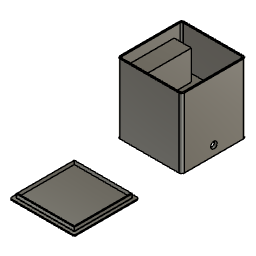
Kinderbastelprojekt, Teo der Topf, v10 (Autodesk Fusion 360 design; units mm, degrees)
part number: Kinderbastelprojekt, Teo der Topf
Autodesk Fusion 360 part; units mm, degrees
sketch "Skizze1" plane through (0, 0, 0) normal (0, 0, 1) x (1, 0, 0)
  line L0 (5, 0) -> (115, 0)
  line L1 (120, 5) -> (120, 115)
  line L2 (115, 120) -> (5, 120)
  line L3 (0, 115) -> (0, 5)
  line L4 (0, 94.8173) -> (30, 94.8173)
  line L5 (30, 94.8173) -> (30, 14.8173)
  line L6 (30, 14.8173) -> (0, 14.8173)
  line L7 (103.4005, 105.0014) -> (105.0005, 105.0014)
  line L8 (105.0005, 105.0014) -> (105.0005, 82.0014)
  line L9 (105.0005, 82.0014) -> (103.4005, 82.0014)
  line L10 (103.4005, 82.0014) -> (103.4005, 105.0014)
  arc A0 (5, 120) -> (0, 115) centre (5, 115) ccw
  arc A1 (120, 115) -> (115, 120) centre (115, 115) ccw
  arc A2 (115, 0) -> (120, 5) centre (115, 5) ccw
  arc A3 (0, 5) -> (5, 0) centre (5, 5) ccw
  point P0 (120, 0)
  point P1 (0, 120)
  dimension "d1" = 120
  dimension "d2" = 120
  dimension "d3" = 30
  dimension "d4" = 80
  dimension "d5" = 1.6
  dimension "d6" = 23
  dimension "d7" = 5
  dimension "d8" = 5
  constraint horizontal L0
  constraint vertical L1
  constraint horizontal L2
  constraint vertical L3
  constraint coincident L3 L4.start
  constraint perpendicular L3 L4
  constraint perpendicular L0 L5
  constraint perpendicular L5 L6
  constraint horizontal L7
  constraint vertical L8
  constraint horizontal L9
  constraint vertical L10
  constraint coincident P1 L2
  constraint coincident P1 L3
  constraint tangent L2 A0
  constraint tangent L3 A0
  constraint tangent L1 A1
  constraint tangent L2 A1
  constraint coincident P0 L0
  constraint coincident P0 L1
  constraint tangent L0 A2
  constraint tangent L1 A2
  constraint equal A1 A2
  constraint coincident origin L0
  constraint coincident origin L3
  constraint tangent L0 A3
  constraint tangent L3 A3
  constraint equal A1 A3
  measures "d1" distance of origin P0
  measures "d2" distance of origin P1
  measures "d3" distance of L4.start L4.end
  measures "d4" distance of L4.end L5.end
  measures "d5" distance of L7.start L7.end
  measures "d6" distance of L7.start L9.end
  measures "d7" radius of A0
  measures "d8" radius of A1
sketch "Skizze2" plane through (0, 0, 0) normal (0, 0, 1) x (1, 0, 0)
  line L0 (5, 115) -> (115, 115)
  line L1 (115, 115) -> (115, 5)
  line L2 (115, 5) -> (5, 5)
  line L3 (5, 5) -> (5, 115)
  constraint horizontal L0
  constraint perpendicular L0 L1
  constraint perpendicular L1 L2
  constraint perpendicular L0 L3
extrude "Extrusion1" add sketch "Skizze1" along normal blind 130 contours L0 L1 L2 L3 L4 L5 L6 A0 A1 A2 A3 makes body 1
extrude "Extrusion2" cut sketch "Skizze2" along normal blind 50 bodies 1
sketch "Skizze3" plane through (0, 0, 130) normal (0, 0, 1) x (-1, 0, 0)
  line L0 (-105.0005, -82.0014) -> (-103.4005, -82.0014)
  line L1 (-103.4005, -82.0014) -> (-103.4005, -105.0014)
  line L2 (-103.4005, -105.0014) -> (-105.0005, -105.0014)
  line L3 (-105.0005, -105.0014) -> (-105.0005, -82.0014)
  arc A0 (0, -5) -> (-5, 0) centre (-5, -5) ccw
  line L4 (-5, 0) -> (-115, 0)
  arc A1 (-115, 0) -> (-120, -5) centre (-115, -5) ccw
  line L5 (-120, -5) -> (-120, -115)
  arc A2 (-120, -115) -> (-115, -120) centre (-115, -115) ccw
  line L6 (-115, -120) -> (-5, -120)
  arc A3 (-5, -120) -> (0, -115) centre (-5, -115) ccw
  line L7 (0, -115) -> (0, -94.8173)
  line L8 (0, -94.8173) -> (-30, -94.8173)
  line L9 (-30, -94.8173) -> (-30, -14.8173)
  line L10 (-30, -14.8173) -> (0, -14.8173)
  line L11 (0, -14.8173) -> (0, -5)
  line L12 (-3, -98) -> (-33, -98)
  line L13 (-33, -98) -> (-33, -14)
  line L14 (-33, -14) -> (-3, -14)
  line L15 (-3, -14) -> (-3, -3)
  line L16 (-3, -3) -> (-117, -3)
  line L17 (-117, -3) -> (-117, -117)
  line L18 (-117, -117) -> (-3, -117)
  line L19 (-3, -117) -> (-3, -98)
  constraint perpendicular L7 L12
  constraint perpendicular L12 L13
  constraint perpendicular L13 L14
  constraint perpendicular L14 L15
  constraint perpendicular L15 L16
  constraint perpendicular L16 L17
  constraint perpendicular L17 L18
  constraint perpendicular L12 L19
extrude "Extrusion3" cut sketch "Skizze3" against normal blind 75 contours L12 L13 L14 L15 L16 L17 L18 L19 bodies 1
sketch "Skizze4" plane through (0, 0, 130) normal (0, 0, 1) x (-1, 0, 0)
  line L0 (-33, -98) -> (-3, -98)
  line L1 (-3, -98) -> (-3, -117)
  line L2 (-3, -117) -> (-117, -117)
  line L3 (-117, -117) -> (-117, -3)
  line L4 (-117, -3) -> (-3, -3)
  line L5 (-3, -3) -> (-3, -14)
  line L6 (-3, -14) -> (-33, -14)
  line L7 (-33, -14) -> (-33, -98)
  arc A0 (0, -5) -> (-5, 0) centre (-5, -5) ccw
  line L8 (-5, 0) -> (-115, 0)
  arc A1 (-115, 0) -> (-120, -5) centre (-115, -5) ccw
  line L9 (-120, -5) -> (-120, -115)
  arc A2 (-120, -115) -> (-115, -120) centre (-115, -115) ccw
  line L10 (-115, -120) -> (-5, -120)
  arc A3 (-5, -120) -> (0, -115) centre (-5, -115) ccw
  line L11 (0, -115) -> (0, -94.8173)
  line L12 (0, -94.8173) -> (-30, -94.8173)
  line L13 (-30, -94.8173) -> (-30, -14.8173)
  line L14 (-30, -14.8173) -> (0, -14.8173)
  line L15 (0, -14.8173) -> (0, -5)
  line L16 (-33, -98) -> (-3, -98)
  line L17 (-3, -98) -> (-3, -14)
  line L18 (-3, -14) -> (-33, -14)
  line L19 (-33, -14) -> (-33, -98)
  constraint horizontal L16
  constraint vertical L17
  constraint horizontal L18
  constraint vertical L19
  constraint coincident L5.end L6.start
  constraint coincident L0.start L7.end
extrude "Extrusion4" add sketch "Skizze4" against normal blind 25 contours L12 L13 L14 L17 bodies 1
sketch "Skizze5" plane through (0, 0, 130) normal (0, 0, 1) x (-1, 0, 0)
  line L0 (-33, -98) -> (-3, -98)
  line L1 (-3, -98) -> (-3, -117)
  line L2 (-3, -117) -> (-117, -117)
  line L3 (-117, -117) -> (-117, -3)
  line L4 (-117, -3) -> (-3, -3)
  line L5 (-3, -3) -> (-3, -14)
  line L6 (-3, -14) -> (-33, -14)
  line L7 (-33, -14) -> (-33, -98)
  arc A0 (0, -5) -> (-5, 0) centre (-5, -5) ccw
  line L8 (-5, 0) -> (-115, 0)
  arc A1 (-115, 0) -> (-120, -5) centre (-115, -5) ccw
  line L9 (-120, -5) -> (-120, -115)
  arc A2 (-120, -115) -> (-115, -120) centre (-115, -115) ccw
  line L10 (-115, -120) -> (-5, -120)
  arc A3 (-5, -120) -> (0, -115) centre (-5, -115) ccw
  line L11 (0, -115) -> (0, -94.8173)
  line L12 (0, -94.8173) -> (-3, -94.8173)
  line L13 (-3, -94.8173) -> (-3, -14.8173)
  line L14 (-3, -14.8173) -> (0, -14.8173)
  line L15 (0, -14.8173) -> (0, -5)
  line L16 (-3, -98) -> (-33, -98)
  line L17 (-33, -98) -> (-33, -14)
  line L18 (-33, -14) -> (-3, -14)
  line L19 (-3, -14) -> (-3, -98)
  constraint horizontal L16
  constraint vertical L17
  constraint horizontal L18
  constraint vertical L19
  constraint coincident L6.end L7.start
  constraint coincident L0.end L1.start
extrude "Extrusion5" cut sketch "Skizze5" against normal blind 23 contours L0 L6 L7 L13 L16 L17 L18 L19 bodies 1
sketch "Skizze6" plane through (117, 0, 0) normal (-1, 0, 0) x (0, -1, 0)
  line L0 (-3, 130) -> (-117, 130)
  line L1 (-117, 130) -> (-117, 55)
  line L2 (-117, 55) -> (-3, 55)
  line L3 (-3, 55) -> (-3, 130)
  line L4 (-95, 130) -> (-15, 130)
  line L5 (-15, 130) -> (-15, 0)
  line L6 (-15, 0) -> (-95, 0)
  line L7 (-95, 0) -> (-95, 130)
  constraint horizontal L4
  constraint vertical L5
  constraint horizontal L6
  constraint vertical L7
  constraint coincident L0 L4.start
sketch "Skizze7" plane through (0, 0, 0) normal (-1, 0, 0) x (0, -1, 0)
  line L0 (-115, 0) -> (-94.8173, 0)
  line L1 (-94.8173, 0) -> (-94.8173, 130)
  line L2 (-94.8173, 130) -> (-115, 130)
  line L3 (-115, 130) -> (-115, 0)
  line L4 (-94.8173, 130) -> (-15, 130)
  line L5 (-15, 130) -> (-15, 0)
  line L6 (-15, 0) -> (-94.8173, 0)
  line L7 (-94.8173, 0) -> (-94.8173, 130)
  constraint horizontal L4
  constraint vertical L5
  constraint horizontal L6
  constraint vertical L7
  constraint coincident L1.end L2.start
sketch "Skizze8" plane through (0, 0, 0) normal (-1, 0, 0) x (0, -1, 0)
  line L0 (-115, 0) -> (-94.8173, 0)
  line L1 (-94.8173, 0) -> (-94.8173, 130)
  line L2 (-94.8173, 130) -> (-115, 130)
  line L3 (-115, 130) -> (-115, 0)
  line L4 (-94.8173, 0) -> (-14.8173, 0)
  line L5 (-14.8173, 0) -> (-14.8173, 50)
  line L6 (-14.8173, 50) -> (-94.8173, 50)
  line L7 (-94.8173, 50) -> (-94.8173, 0)
  dimension "d19" = 80
  dimension "d20" = 50
  constraint horizontal L4
  constraint vertical L5
  constraint horizontal L6
  constraint vertical L7
  constraint coincident L0.end L1.start
  measures "d19" distance of L0.end L4.end
  measures "d20" distance of L0.end L6.end
extrude "Extrusion6" add sketch "Skizze8" against normal blind 5 contours L1 L4 L5 L6 L7 bodies 1
sketch "Skizze9" plane through (0, 0, 0) normal (-1, 0, 0) x (0, -1, 0)
  line L0 (-115, 0) -> (-5, 0)
  line L1 (-5, 0) -> (-5, 130)
  line L2 (-5, 130) -> (-14.8173, 130)
  line L3 (-14.8173, 130) -> (-14.8173, 50)
  line L4 (-14.8173, 50) -> (-94.8173, 50)
  line L5 (-94.8173, 50) -> (-94.8173, 130)
  line L6 (-94.8173, 130) -> (-115, 130)
  line L7 (-115, 130) -> (-115, 0)
  line L8 (-94.8173, 130) -> (-14.8173, 130)
  line L9 (-14.8173, 130) -> (-14.8173, 105)
  line L10 (-14.8173, 105) -> (-94.8173, 105)
  line L11 (-94.8173, 105) -> (-94.8173, 130)
  dimension "d23" = 80
  dimension "d24" = 25
  constraint horizontal L8
  constraint vertical L9
  constraint horizontal L10
  constraint vertical L11
  constraint coincident L5.end L6.start
  measures "d23" distance of L5.end L2.end
  measures "d24" distance of L5.end L10.end
extrude "Extrusion7" add sketch "Skizze9" against normal blind 3 contours L3 L5 L8 L9 L10 L11 bodies 1
sketch "Skizze10" plane through (0, 0, 0) normal (-1, 0, 0) x (0, -1, 0)
  line L0 (-14.8173, 105) -> (-14.8173, 50)
  line L1 (-14.8173, 50) -> (-94.8173, 50)
  line L2 (-94.8173, 50) -> (-94.8173, 105)
  line L3 (-94.8173, 105) -> (-14.8173, 105)
  line L4 (-5, 130) -> (-115, 130)
  line L5 (-115, 130) -> (-115, 0)
  line L6 (-115, 0) -> (-5, 0)
  line L7 (-5, 0) -> (-5, 130)
  line L8 (-94.8173, 105) -> (-14.8173, 105)
  line L9 (-14.8173, 105) -> (-14.8173, 50)
  line L10 (-14.8173, 50) -> (-94.8173, 50)
  line L11 (-94.8173, 50) -> (-94.8173, 105)
  constraint horizontal L8
  constraint vertical L9
  constraint horizontal L10
  constraint vertical L11
  constraint coincident L1 L0.end
  constraint coincident L0 L1.start
  constraint coincident L2.end L3.start
extrude "Extrusion8" add sketch "Skizze10" against normal blind 2 contours L0 L1 L2 L3 L8 L9 L10 L11 bodies 1
move_face "Fläche verschieben1" by (0, 5, 0) 3 faces at (11.3333, 41.484, 105) (30, 68.1506, 68.3333) (12.3333, 14.8173, 86.6667) on bodies 1
move_face "Fläche verschieben2" by (0, 5, 0) 1 faces at (23, 42, 107) on bodies 1
move_face "Fläche verschieben3" by (0, 10, 0) 1 faces at (20.6667, 69.8173, 105) on bodies 1
sketch "Skizze11" plane through (0, 94.8173, 0) normal (0, -1, 0) x (1, 0, 0)
  line L0 (2, 105) -> (2, 50)
  line L1 (2, 50) -> (5, 50)
  line L2 (5, 50) -> (30, 50)
  line L3 (30, 50) -> (30, 105)
  line L4 (30, 105) -> (2, 105)
extrude "Extrusion9" cut sketch "Skizze11" against normal blind 1 bodies 1
move_face "Flächen versetzen1" offset -1 1 faces at (12.3333, 19.8173, 86.6667) on bodies 1
extrude "Extrusion10" add 1 faces at (13, 98, 89.6667) along direction (0, -1, 0) blind 2.338 on bodies 1 bodies 1
move_face "Fläche verschieben4" by (0, 5, 0) 1 faces at (13, 42, 107) on bodies 1
move_face "Fläche verschieben5" by (0, 5, 0) 2 faces at (33, 42, 72.3333) (13, 42, 107) on bodies 1
delete_face "Fläche löschen1" 1 faces at (11.6667, 44.4322, 105) on bodies 1
delete_face "Fläche löschen2" 1 faces at (13, 98, 89.6667) on bodies 1
delete_face "Fläche löschen3" 1 faces at (13, 14, 72.3333) on bodies 1
delete_face "Fläche löschen4" 1 faces at (2, 44.484, 103.3333) on bodies 1
sketch "Skizze12" plane through (0, 0, 107) normal (0, 0, 1) x (-1, 0, 0)
  line L0 (-33, -3) -> (-33, -117)
  line L1 (-33, -117) -> (-3, -117)
  line L2 (-3, -117) -> (-3, -95.8173)
  line L3 (-3, -95.8173) -> (-3, -95.662)
  line L4 (-3, -95.662) -> (-30, -95.662)
  line L5 (-30, -95.662) -> (-30, -18.8173)
  line L6 (-30, -18.8173) -> (-3, -18.8173)
  line L7 (-3, -18.8173) -> (-3, -3)
  line L8 (-3, -3) -> (-33, -3)
  line L9 (-33, -3) -> (-3, -3)
  line L10 (-3, -3) -> (-3, -117)
  line L11 (-3, -117) -> (-33, -117)
  line L12 (-33, -117) -> (-33, -3)
  constraint horizontal L9
  constraint vertical L10
  constraint horizontal L11
  constraint vertical L12
  constraint coincident L1.end L2.start
  constraint coincident L0.start L8.end
extrude "Extrusion11" cut sketch "Skizze12" against normal blind 52 bodies 1
sketch "Skizze13" plane through (0, 0, 0) normal (0, 0, 1) x (1, 0, 0)
  line L0 (30, 96, 130) -> (3, 96, 130)
  line L1 (3, 96, 130) -> (3, 19, 130)
  line L2 (3, 19, 130) -> (30, 19, 130)
  line L3 (30, 19, 130) -> (30, 96, 130)
sketch "Skizze14" plane through (0, 0, 50) normal (0, 0, 1) x (-1, 0, 0)
  line L0 (-5, -95.8173) -> (0, -95.8173)
  line L1 (0, -95.8173) -> (0, -18.8173)
  line L2 (0, -18.8173) -> (-5, -18.8173)
  line L3 (-5, -18.8173) -> (-5, -95.8173)
  line L4 (0, -95.8173) -> (-5, -95.8173)
  line L5 (-5, -95.8173) -> (-5, -18.8173)
  line L6 (-5, -18.8173) -> (0, -18.8173)
  line L7 (0, -18.8173) -> (0, -95.8173)
  constraint horizontal L4
  constraint vertical L5
  constraint horizontal L6
  constraint vertical L7
  constraint coincident L2.end L3.start
  constraint coincident L0.end L1.start
extrude "Extrusion12" add sketch "Skizze14" along normal blind 80 bodies 1
sketch "Skizze15" plane through (0, 0, 55) normal (0, 0, 1) x (-1, 0, 0)
  line L0 (-103.4005, -105.0014) -> (-105.0005, -105.0014)
  line L1 (-105.0005, -105.0014) -> (-105.0005, -82.0014)
  line L2 (-105.0005, -82.0014) -> (-103.4005, -82.0014)
  line L3 (-103.4005, -82.0014) -> (-103.4005, -105.0014)
  line L4 (-3, -3) -> (-117, -3)
  line L5 (-117, -3) -> (-117, -117)
  line L6 (-117, -117) -> (-3, -117)
  line L7 (-3, -117) -> (-3, -95.8173)
  line L8 (-3, -95.8173) -> (-5, -95.8173)
  line L9 (-5, -95.8173) -> (-30, -95.8173)
  line L10 (-30, -95.8173) -> (-30, -18.8173)
  line L11 (-30, -18.8173) -> (-5, -18.8173)
  line L12 (-5, -18.8173) -> (-3, -18.8173)
  line L13 (-3, -18.8173) -> (-3, -3)
  line L14 (-3, -95.8173) -> (-30, -95.8173)
  line L15 (-30, -95.8173) -> (-30, -18.8173)
  line L16 (-30, -18.8173) -> (-3, -18.8173)
  line L17 (-3, -18.8173) -> (-3, -95.8173)
  constraint horizontal L14
  constraint vertical L15
  constraint horizontal L16
  constraint vertical L17
  constraint coincident L10.end L11.start
  constraint coincident L7.end L8.start
sketch "Skizze16" plane through (0, 0, 50) normal (0, 0, -1) x (1, 0, 0)
  line L0 (5, -115) -> (115, -115)
  line L1 (115, -115) -> (115, -5)
  line L2 (115, -5) -> (5, -5)
  line L3 (5, -5) -> (5, -18.8173)
  line L4 (5, -18.8173) -> (30, -18.8173)
  line L5 (30, -18.8173) -> (30, -95.8173)
  line L6 (30, -95.8173) -> (5, -95.8173)
  line L7 (5, -95.8173) -> (5, -115)
  line L8 (105.0005, -82.0014) -> (105.0005, -105.0014)
  line L9 (105.0005, -105.0014) -> (103.4005, -105.0014)
  line L10 (103.4005, -105.0014) -> (103.4005, -82.0014)
  line L11 (103.4005, -82.0014) -> (105.0005, -82.0014)
  line L12 (30, -95.8173) -> (5, -95.8173)
  line L13 (5, -95.8173) -> (5, -18.8173)
  line L14 (5, -18.8173) -> (30, -18.8173)
  line L15 (30, -18.8173) -> (30, -95.8173)
  constraint horizontal L12
  constraint vertical L13
  constraint horizontal L14
  constraint vertical L15
  constraint coincident L3.end L4.start
  constraint coincident L5.end L6.start
extrude "Extrusion13" add sketch "Skizze16" against normal blind 5 separate body contours L4 L5 L6 L12 L13 L14 L15 makes body 2
sketch "Skizze17" plane through (5, 0, 0) normal (1, 0, 0) x (0, 1, 0)
  line L0 (5, 0) -> (115, 0)
  line L1 (115, 0) -> (115, 50)
  line L2 (115, 50) -> (95.8173, 50)
  line L3 (95.8173, 50) -> (95.8173, 55)
  line L4 (95.8173, 55) -> (95.8173, 130)
  line L5 (95.8173, 130) -> (18.8173, 130)
  line L6 (18.8173, 130) -> (18.8173, 55)
  line L7 (18.8173, 55) -> (18.8173, 50)
  line L8 (18.8173, 50) -> (5, 50)
  line L9 (5, 50) -> (5, 0)
  line L10 (18.8173, 130) -> (95.8173, 130)
  line L11 (95.8173, 130) -> (95.8173, 55)
  line L12 (95.8173, 55) -> (18.8173, 55)
  line L13 (18.8173, 55) -> (18.8173, 130)
  constraint horizontal L10
  constraint vertical L11
  constraint horizontal L12
  constraint vertical L13
  constraint coincident L3.end L4.start
  constraint coincident L5.end L6.start
extrude "Extrusion14" cut sketch "Skizze17" against normal blind 2 contours L4 L5 L6 L10 L11 L12 L13 bodies 1
sketch "Skizze18" plane through (0, 0, 50) normal (0, 0, -1) x (1, 0, 0)
  line L0 (5, -115) -> (115, -115)
  line L1 (115, -115) -> (115, -5)
  line L2 (115, -5) -> (5, -5)
  line L3 (5, -5) -> (5, -18.8173)
  line L4 (5, -18.8173) -> (30, -18.8173)
  line L5 (5, -95.8173) -> (5, -115)
  line L6 (105.0005, -82.0014) -> (105.0005, -105.0014)
  line L7 (105.0005, -105.0014) -> (103.4005, -105.0014)
  line L8 (103.4005, -105.0014) -> (103.4005, -82.0014)
  line L9 (103.4005, -82.0014) -> (105.0005, -82.0014)
  line L10 (2.0083, -103.0001) -> (35.0083, -103.0001)
  line L11 (35.0083, -103.0001) -> (35.0083, -17.0001)
  line L12 (35.0083, -17.0001) -> (2.0083, -17.0001)
  line L13 (2.0083, -17.0001) -> (2.0083, -103.0001)
  dimension "d44" = 33
  dimension "d45" = 86
  constraint horizontal L10
  constraint vertical L11
  constraint horizontal L12
  constraint vertical L13
  measures "d44" distance of L10.start L10.end
  measures "d45" distance of L10.start L12.end
extrude "Extrusion15" cut sketch "Skizze18" against normal blind 60 contours L10 L11 L12 L13 bodies 1 2
sketch "Skizze19" plane through (0, 0, 55) normal (0, 0, 1) x (-1, 0, 0)
  line L0 (-35.0083, -17.0001) -> (-3, -17.0001)
  line L1 (-3, -17.0001) -> (-3, -3)
  line L2 (-3, -3) -> (-117, -3)
  line L3 (-117, -3) -> (-117, -117)
  line L4 (-117, -117) -> (-3, -117)
  line L5 (-3, -117) -> (-3, -103.0001)
  line L6 (-3, -103.0001) -> (-35.0083, -103.0001)
  line L7 (-35.0083, -103.0001) -> (-35.0083, -17.0001)
  line L8 (-103.4005, -105.0014) -> (-105.0005, -105.0014)
  line L9 (-105.0005, -105.0014) -> (-105.0005, -82.0014)
  line L10 (-105.0005, -82.0014) -> (-103.4005, -82.0014)
  line L11 (-103.4005, -82.0014) -> (-103.4005, -105.0014)
  line L12 (-3, -17.0001) -> (-3, -14.0001)
  line L13 (-3, -14.0001) -> (-38, -14.0001)
  line L14 (-38, -14.0001) -> (-38, -106)
  line L15 (-38, -106) -> (-3, -106)
  line L16 (-3, -103.0001) -> (-3, -106)
  dimension "d48" = 3
  constraint coincident L0.end L1.start
  constraint coincident L1 L12.end
  constraint perpendicular L7 L13
  constraint perpendicular L13 L14
  constraint coincident L5 L15.end
  constraint perpendicular L5 L15
  constraint coincident L5.end L6.start
  measures "d48" distance of L0.end L12.end
sketch "Skizze20" plane through (0, 0, 55) normal (0, 0, 1) x (-1, 0, 0)
  line L0 (-35.0083, -17.0001) -> (-3, -17.0001)
  line L1 (-3, -17.0001) -> (-3, -3)
  line L2 (-3, -3) -> (-117, -3)
  line L3 (-117, -3) -> (-117, -117)
  line L4 (-117, -117) -> (-3, -117)
  line L5 (-3, -117) -> (-3, -103.0001)
  line L6 (-3, -103.0001) -> (-35.0083, -103.0001)
  line L7 (-35.0083, -103.0001) -> (-35.0083, -17.0001)
  line L8 (-103.4005, -105.0014) -> (-105.0005, -105.0014)
  line L9 (-105.0005, -105.0014) -> (-105.0005, -82.0014)
  line L10 (-105.0005, -82.0014) -> (-103.4005, -82.0014)
  line L11 (-103.4005, -82.0014) -> (-103.4005, -105.0014)
  line L12 (-3, -103.0001) -> (-3, -101)
  line L13 (-3, -101) -> (-33, -101)
  line L14 (-33, -101) -> (-33, -19)
  line L15 (-33, -19) -> (-5, -19)
  line L16 (-5, -19) -> (-5, -17.0001)
  line L17 (-35.0083, -17.0001) -> (-35.0083, -103.0001)
  line L18 (-3, -103.0001) -> (-3, -101)
  constraint coincident L5.end L6.start
  constraint perpendicular L6 L12
  constraint perpendicular L7 L13
  constraint perpendicular L0 L14
  constraint perpendicular L14 L15
  constraint coincident L0 L16.end
  constraint perpendicular L0 L16
  constraint coincident L0.start L7.end
  constraint coincident L6.end L7.start
sketch "Skizze21" plane through (0, 0, 55) normal (0, 0, 1) x (-1, 0, 0)
  line L0 (-35.0083, -17.0001) -> (-3, -17.0001)
  line L1 (-3, -17.0001) -> (-3, -3)
  line L2 (-3, -3) -> (-117, -3)
  line L3 (-117, -3) -> (-117, -117)
  line L4 (-117, -117) -> (-3, -117)
  line L5 (-3, -117) -> (-3, -103.0001)
  line L6 (-3, -103.0001) -> (-35.0083, -103.0001)
  line L7 (-35.0083, -103.0001) -> (-35.0083, -17.0001)
  line L8 (-103.4005, -105.0014) -> (-105.0005, -105.0014)
  line L9 (-105.0005, -105.0014) -> (-105.0005, -82.0014)
  line L10 (-105.0005, -82.0014) -> (-103.4005, -82.0014)
  line L11 (-103.4005, -82.0014) -> (-103.4005, -105.0014)
  line L12 (0.0095, -17.0001) -> (-35.0083, -17.0001)
  line L13 (-35.0083, -17.0001) -> (-35.0083, -103.0001)
  line L14 (-0.0568, -103.0001) -> (0.0095, -17.0001)
  line L15 (-0.0568, -19.1107) -> (-33.0568, -19.0853)
  line L16 (-33.0568, -19.0853) -> (-33.12, -101.0852)
  line L17 (-33.12, -101.0852) -> (-0.0553, -101.1107)
  dimension "d49" = 33
  dimension "d50" = 82
  constraint coincident L0.start L7.end
  constraint perpendicular L7 L12
  constraint coincident L6.end L7.start
  constraint perpendicular L14 L15
  constraint perpendicular L15 L16
  constraint coincident L14 L17.end
  constraint perpendicular L14 L17
  measures "d49" distance of L15.start L15.end
  measures "d50" distance of L15.end L16.end
sketch "Skizze22" plane through (2.0083, 0, 0) normal (1, 0, 0) x (0, 1, 0)
  line L0 (17.0001, 50) -> (103.0001, 50)
  line L1 (103.0001, 50) -> (103.0001, 110)
  line L2 (103.0001, 110) -> (17.0001, 110)
  line L3 (17.0001, 110) -> (17.0001, 50)
  line L4 (19, 54) -> (17.0001, 54)
  line L5 (17.0001, 110) -> (103.0001, 110)
  line L6 (104, 54) -> (102, 54)
  line L7 (102, 54) -> (102, 108)
  line L8 (102, 108) -> (19, 108)
  line L9 (19, 108) -> (19, 54)
  constraint coincident L3 L4.end
  constraint perpendicular L3 L4
  constraint coincident L2.end L3.start
  constraint coincident L1.end L2.start
  constraint perpendicular L1 L6
  constraint perpendicular L6 L7
  constraint perpendicular L3 L8
  constraint perpendicular L4 L9
sketch "Skizze23" plane through (0, 0, 55) normal (0, 0, 1) x (-1, 0, 0)
  line L0 (-35.0083, -17.0001) -> (-3, -17.0001)
  line L1 (-3, -17.0001) -> (-3, -3)
  line L2 (-3, -3) -> (-117, -3)
  line L3 (-117, -3) -> (-117, -117)
  line L4 (-117, -117) -> (-3, -117)
  line L5 (-3, -117) -> (-3, -103.0001)
  line L6 (-3, -103.0001) -> (-35.0083, -103.0001)
  line L7 (-35.0083, -103.0001) -> (-35.0083, -17.0001)
  line L8 (-103.4005, -105.0014) -> (-105.0005, -105.0014)
  line L9 (-105.0005, -105.0014) -> (-105.0005, -82.0014)
  line L10 (-105.0005, -82.0014) -> (-103.4005, -82.0014)
  line L11 (-103.4005, -82.0014) -> (-103.4005, -105.0014)
  line L12 (0, -17) -> (0, -19)
  line L13 (0, -19) -> (-33, -19)
  line L14 (-33, -19) -> (-33, -101)
  line L15 (-33, -101) -> (0, -101)
  line L16 (0, -101) -> (0, -103)
  line L17 (0, -103) -> (-35.0083, -103.0001)
  line L18 (-35.0083, -17.0001) -> (0, -17)
  constraint vertical L12
  constraint perpendicular L7 L13
  constraint perpendicular L6 L14
  constraint perpendicular L14 L15
  constraint perpendicular L13 L16
  constraint coincident L6.end L7.start
  constraint coincident L0.start L7.end
sketch "Skizze24" plane through (0, 0, 55) normal (0, 0, 1) x (-1, 0, 0)
  line L0 (-35.0083, -17.0001) -> (-3, -17.0001)
  line L1 (-3, -17.0001) -> (-3, -3)
  line L2 (-3, -3) -> (-117, -3)
  line L3 (-117, -3) -> (-117, -117)
  line L4 (-117, -117) -> (-3, -117)
  line L5 (-3, -117) -> (-3, -103.0001)
  line L6 (-3, -103.0001) -> (-35.0083, -103.0001)
  line L7 (-35.0083, -103.0001) -> (-35.0083, -17.0001)
  line L8 (-103.4005, -105.0014) -> (-105.0005, -105.0014)
  line L9 (-105.0005, -105.0014) -> (-105.0005, -82.0014)
  line L10 (-105.0005, -82.0014) -> (-103.4005, -82.0014)
  line L11 (-103.4005, -82.0014) -> (-103.4005, -105.0014)
  line L12 (-35.0083, -103.0001) -> (-0.0083, -103.0001)
  line L13 (-0.0083, -103.0001) -> (-0.0083, -17.0001)
  line L14 (-0.0083, -17.0001) -> (-35.0083, -17.0001)
  line L15 (-35.0083, -17.0001) -> (-35.0083, -103.0001)
  dimension "d51" = 35
  dimension "d52" = 86
  constraint horizontal L12
  constraint vertical L13
  constraint horizontal L14
  constraint vertical L15
  constraint coincident L6.end L7.start
  measures "d51" distance of L6.end L12.end
  measures "d52" distance of L6.end L0.start
sketch "Skizze25" plane through (0, 0, 50) normal (0, 0, -1) x (1, 0, 0)
  line L0 (105.0005, -82.0014) -> (105.0005, -105.0014)
  line L1 (105.0005, -105.0014) -> (103.4005, -105.0014)
  line L2 (103.4005, -105.0014) -> (103.4005, -82.0014)
  line L3 (103.4005, -82.0014) -> (105.0005, -82.0014)
  line L4 (5, -17.0001) -> (35.0083, -17.0001)
  line L5 (35.0083, -17.0001) -> (35.0083, -103.0001)
  line L6 (35.0083, -103.0001) -> (5, -103.0001)
  line L7 (5, -103.0001) -> (5, -115)
  line L8 (5, -115) -> (115, -115)
  line L9 (115, -115) -> (115, -5)
  line L10 (115, -5) -> (5, -5)
  line L11 (5, -5) -> (5, -17.0001)
  line L12 (0, -101) -> (33, -101)
  line L13 (33, -101) -> (33, -19)
  line L14 (33, -19) -> (0, -19)
  line L15 (0, -19) -> (0, -17.0001)
  line L16 (0, -17.0001) -> (35.0083, -17.0001)
  line L17 (35.0083, -103.0001) -> (0, -103.0001)
  line L18 (0, -103.0001) -> (0, -101)
  constraint perpendicular L7 L12
  constraint perpendicular L4 L13
  constraint perpendicular L13 L14
  constraint perpendicular L14 L15
  constraint coincident L4.end L5.start
  constraint perpendicular L5 L16
  constraint coincident L5.end L6.start
  constraint perpendicular L7 L17
  constraint perpendicular L12 L18
extrude "Extrusion16" add sketch "Skizze25" against normal blind 60 contours L4 L5 L6 L12 L13 L14 L15 L16 L17 L18 bodies 1 2
sketch "Skizze26" plane through (0, 0, 110) normal (0, 0, 1) x (-1, 0, 0)
  line L0 (-3, -19) -> (-3, -17.0001)
  line L1 (-3, -17.0001) -> (-35.0083, -17.0001)
  line L2 (-35.0083, -17.0001) -> (-35.0083, -103.0001)
  line L3 (-35.0083, -103.0001) -> (-3, -103.0001)
  line L4 (-3, -103.0001) -> (-3, -101)
  line L5 (-3, -101) -> (-33, -101)
  line L6 (-33, -101) -> (-33, -19)
  line L7 (-33, -19) -> (-3, -19)
  line L8 (-35.0083, -103.0001) -> (-0.0083, -103.0001)
  line L9 (-0.0083, -103.0001) -> (-0.0083, -17.0001)
  line L10 (-0.0083, -17.0001) -> (-35.0083, -17.0001)
  line L11 (-35.0083, -17.0001) -> (-35.0083, -103.0001)
  dimension "d55" = 35
  dimension "d56" = 86
  constraint horizontal L8
  constraint vertical L9
  constraint horizontal L10
  constraint vertical L11
  constraint coincident L2.end L3.start
  measures "d55" distance of L2.end L8.end
  measures "d56" distance of L2.end L1.end
extrude "Extrusion17" add sketch "Skizze26" against normal blind 2 contours L0 L4 L5 L6 L7 L8 L9 L10 bodies 1
sketch "Skizze27" plane through (0, 0, 0) normal (-1, 0, 0) x (0, -1, 0)
  line L0 (-5, 0) -> (-5, 130)
  line L1 (-5, 130) -> (-115, 130)
  line L2 (-115, 130) -> (-115, 0)
  line L3 (-115, 0) -> (-5, 0)
  circle A0 centre (-60, 85) radius 20
  point P0 (-60, 85)
  dimension "d59" = 40
  constraint coincident P0 A0.centre
  measures "d59" diameter of A0
extrude "Extrusion18" cut sketch "Skizze27" against normal blind 3 contours A0 bodies 1
fillet "Abrundung1" radius 3 1 edges at (117, 117, 92.5) on bodies 1
fillet "Abrundung2" radius 3 1 edges at (117, 3, 92.5) on bodies 1
fillet "Abrundung3" radius 3 1 edges at (3, 117, 92.5) on bodies 1
fillet "Abrundung4" radius 3 1 edges at (3, 3, 92.5) on bodies 1
fillet "Abrundung5" radius 1 1 faces at (1, 46.2724, 130) on bodies 1
fillet "Abrundung6" radius 0.5 1 edges at (0, 78.6465, 92.2323) on bodies 1
sketch "Skizze28" plane through (0, 0, 0) normal (0, 0, -1) x (1, 0, 0)
  line L0 (0, -5) -> (0, -115)
  arc A0 (0, -115) -> (5, -120) centre (5, -115) ccw
  line L1 (5, -120) -> (115, -120)
  arc A1 (115, -120) -> (120, -115) centre (115, -115) ccw
  line L2 (120, -115) -> (120, -5)
  arc A2 (120, -5) -> (115, 0) centre (115, -5) ccw
  line L3 (115, 0) -> (5, 0)
  arc A3 (5, 0) -> (0, -5) centre (5, -5) ccw
  line L4 (5, -115) -> (5, -5)
  line L5 (5, -5) -> (115, -5)
  line L6 (115, -5) -> (115, -115)
  line L7 (115, -115) -> (5, -115)
  line L8 (-53, 29.8241, -10.0084) -> (-167, 29.8241, -10.0084)
  line L9 (-170, 32.8241, -10.0084) -> (-170, 146.8241, -10.0084)
  line L10 (-167, 149.8241, -10.0084) -> (-53, 149.8241, -10.0084)
  line L11 (-50, 146.8241, -10.0084) -> (-50, 32.8241, -10.0084)
  arc A4 through (-53, 29.8241, -10.0084) (-50.8787, 30.7027, -10.0084) (-50, 32.8241, -10.0084)
  arc A5 through (-170, 32.8241, -10.0084) (-169.1213, 30.7027, -10.0084) (-167, 29.8241, -10.0084)
  arc A6 through (-167, 149.8241, -10.0084) (-169.1213, 148.9454, -10.0084) (-170, 146.8241, -10.0084)
  arc A7 through (-50, 146.8241, -10.0084) (-50.8787, 148.9454, -10.0084) (-53, 149.8241, -10.0084)
  line L12 (-56.0002, 35.8243, -10.0084) -> (-164.0002, 35.8243, -10.0084)
  line L13 (-164.0002, 35.8243, -10.0084) -> (-164.0002, 143.8243, -10.0084)
  line L14 (-164.0002, 143.8243, -10.0084) -> (-56.0002, 143.8243, -10.0084)
  line L15 (-56.0002, 143.8243, -10.0084) -> (-56.0002, 35.8243, -10.0084)
  point P0 (-50, 29.8241)
  point P1 (-170, 29.8241)
  point P2 (-50, 149.8241)
  dimension "d74" = 120
  dimension "d75" = 120
  dimension "d76" = 3
  dimension "d77" = 108
  dimension "d78" = 108
  measures "d74" distance of P0 P1
  measures "d75" distance of P0 P2
extrude "Extrusion19" add sketch "Skizze28" along normal blind 10 separate body contours L8 L9 L10 L11 A4 A5 A6 A7 | L12 L13 L14 L15 in plane through (0, 0, 10.0084) normal (0, 0, -1) makes body 3
extrude "Extrusion20" cut sketch "Skizze28" along normal blind 8 contours L8 L9 L10 L11 A4 A5 A6 A7 in plane through (0, 0, 10.0084) normal (0, 0, -1) bodies 3
sketch "Skizze29" plane through (0, 0, 10.0084) normal (0, 0, -1) x (1, 0, 0)
  line L0 (-58, -8) -> (-162, -8)
  line L1 (-162, -8) -> (-162, -112)
  line L2 (-162, -112) -> (-58, -112)
  line L3 (-58, -112) -> (-58, -8)
  dimension "d83" = 104
  dimension "d84" = 104
  constraint horizontal L0
  constraint vertical L1
  constraint horizontal L2
  constraint vertical L3
  measures "d83" distance of L0.start L0.end
  measures "d84" distance of L0.start L2.end
extrude "Extrusion21" cut sketch "Skizze29" along normal blind 8 bodies 3
fillet "Abrundung7" radius 1 4 edges at (-56.0002, -89.8243, 10.0084) (-110.0002, -143.8243, 10.0084) (-164.0002, -89.8243, 10.0084) (-110.0002, -35.8243, 10.0084) on bodies 3
sketch "Skizze30" plane through (0, 0, 0) normal (-1, 0, 0) x (0, -1, 0)
  line L0 (-5, 129) -> (-115, 129)
  line L1 (-115, 129) -> (-115, 0)
  line L2 (-115, 0) -> (-5, 0)
  line L3 (-5, 0) -> (-5, 129)
  circle A0 centre (-60, 85) radius 20.5
extrude "Extrusion22" cut 1 faces at (-92.3335, -107.491, 10.0084) along direction (0, 0, -1) blind 7 on bodies 3 bodies 3
sketch "Skizze31" plane through (2.0083, 0, 0) normal (1, 0, 0) x (0, 1, 0)
  circle A0 centre (60, 85) radius 20
  line L0 (101, 108) -> (19, 108)
  line L1 (19, 108) -> (19, 50)
  line L2 (19, 50) -> (101, 50)
  line L3 (101, 50) -> (101, 108)
  line L4 (101, 62) -> (19, 62)
  line L5 (19, 62) -> (19, 63)
  line L6 (19, 63) -> (101, 63)
  line L7 (101, 63) -> (101, 62)
  constraint horizontal L4
  constraint vertical L5
  constraint horizontal L6
  constraint vertical L7
  constraint coincident L1 L5.end
  constraint coincident L3 L4.start
extrude "Extrusion23" add sketch "Skizze31" along normal blind 5 contours L1 L3 L4 L5 L6 L7 bodies 1
sketch "Skizze32" plane through (0, 0, 62) normal (0, 0, -1) x (1, 0, 0)
  line L0 (2.0083, -19) -> (2.0083, -101)
  line L1 (2.0083, -101) -> (7.0083, -101)
  line L2 (7.0083, -101) -> (7.0083, -19)
  line L3 (7.0083, -19) -> (2.0083, -19)
  line L4 (7.0083, -25.0002) -> (2.0083, -25.0002)
  line L5 (2.0083, -25.0002) -> (2.0083, -95.0002)
  line L6 (2.0083, -95.0002) -> (7.0083, -95.0002)
  line L7 (7.0083, -95.0002) -> (7.0083, -25.0002)
  dimension "d93" = 70
  constraint horizontal L4
  constraint vertical L5
  constraint horizontal L6
  constraint vertical L7
  constraint coincident L2 L4.start
  measures "d93" distance of L4.start L6.end
extrude "Extrusion24" cut sketch "Skizze32" against normal blind 1 contours L0 L2 L4 L5 L6 L7 bodies 1
move_body "Verschieben1" bodies 3 to x (1, 0, 0) y (0, 1, 0) z (0, 0, 1) at (170, -50, 0)
sketch "Skizze33" plane through (115, 0, 0) normal (-1, 0, 0) x (0, -1, 0)
  line L0 (-115, 0) -> (-5, 0)
  line L1 (-5, 0) -> (-5, 50)
  line L2 (-5, 50) -> (-115, 50)
  line L3 (-115, 50) -> (-115, 0)
  line L4 (-15, 40) -> (-30, 40)
  line L5 (-30, 40) -> (-30, 20)
  line L6 (-30, 20) -> (-15, 20)
  line L7 (-15, 20) -> (-15, 40)
  dimension "d96" = 15
  dimension "d97" = 20
  constraint horizontal L4
  constraint vertical L5
  constraint horizontal L6
  constraint vertical L7
  measures "d96" distance of L4.start L4.end
  measures "d97" distance of L4.start L6.end
extrude "Extrusion25" cut sketch "Skizze33" against normal blind 3 contours L4 L5 L6 L7 bodies 1
sketch "Skizze34" plane through (118, 0, 0) normal (-1, 0, 0) x (0, -1, 0)
  line L0 (-15, 20) -> (-15, 40)
  line L1 (-15, 40) -> (-30, 40)
  line L2 (-30, 40) -> (-30, 20)
  line L3 (-30, 20) -> (-15, 20)
  circle A0 centre (-28, 38) radius 1.4
  point P0 (-28, 38)
  dimension "d100" = 2.8
  constraint coincident P0 A0.centre
  measures "d100" diameter of A0
extrude "Extrusion26" add sketch "Skizze34" along normal blind 3 contours A0 bodies 1
move_face "Fläche verschieben6" to x (1, 0, 0) y (0, 1, 0) z (0, 0, 1) at (0, -0.5, -0.5) 2 faces at (115, 28.4297, 37.6455) (116, 26.8054, 37.27) on bodies 1
move_face "Fläche verschieben7" to x (1, 0, 0) y (0, 1, 0) z (0, 0, 1) at (0, -0.5, -0.5) 2 faces at (115, 27.9297, 37.1455) (116, 26.3054, 36.77) on bodies 1
sketch "Skizze35" plane through (115, 0, 0) normal (-1, 0, 0) x (0, -1, 0)
  line L0 (-30, 40) -> (-15, 40)
  line L1 (-15, 40) -> (-15, 20)
  line L2 (-15, 20) -> (-30, 20)
  line L3 (-30, 20) -> (-30, 40)
  line L4 (-115, 0) -> (-5, 0)
  line L5 (-5, 0) -> (-5, 50)
  line L6 (-5, 50) -> (-115, 50)
  line L7 (-115, 50) -> (-115, 0)
  circle A0 centre (-60, 17.5427) radius 6
  dimension "d104" = 12
  measures "d104" diameter of A0
extrude "Extrusion27" cut sketch "Skizze35" against normal blind 5 contours A0 bodies 1
